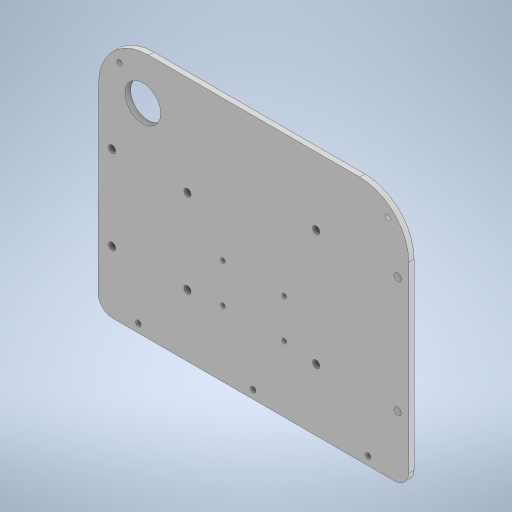
# Autodesk Inventor part: Final_Back_Cover_1
Saved by Autodesk Inventor 2023.5 (Build 275446020, 446B)
## iProperties
Created: 2025-04-13
Part Number: Final_Back_Cover_1
Material: Generic
Document SubType Name: Modeling
Designer: Lucky
Density: 1 g/cm^3
Appearance: Default
Author: Lucky
Autodesk Inventor part; units mm, degrees
ref_plane "YZ Plane" through (0, 0, 0) normal (1, 0, 0) x (0, 1, 0)
ref_plane "XZ Plane" through (0, 0, 0) normal (0, 1, 0) x (-1, 0, 0)
ref_plane "XY Plane" through (0, 0, 0) normal (0, 0, 1) x (1, 0, 0)
sketch "Sketch1" plane through (0, 0, 0) normal (0, 0, 1) x (1, 0, 0)
  arc A0 (-85.6258, 79.4796) -> (-116.0775, 49.6172) centre (-86.1702, 49.5773) ccw
  line L0 (-85.6258, 79.4796) -> (33.3305, 79.4959)
  arc A1 (63.2389, 49.5916) -> (33.3305, 79.4959) centre (33.3346, 49.5916) ccw
  line L1 (63.2389, -50.9075) -> (63.2389, 49.5916)
  line L2 (63.2389, 49.5916) -> (63.2389, -53.5021)
  line L3 (-116.0775, 49.6172) -> (-116.3855, -51.7391)
  line L4 (-116.0775, 49.6172) -> (-116.0775, -50.4074)
  arc A2 (-116.3855, -51.7391) -> (-106.0129, -63.5021) centre (-106.0129, -53.0473) ccw
  line L5 (-106.0129, -63.5021) -> (53.2389, -63.5021)
  arc A3 (53.2389, -63.5021) -> (63.2389, -53.5021) centre (53.2389, -53.5021) ccw
  arc A4 (-86.7039, 77.4795) -> (-114.0775, 49.6129) centre (-86.1702, 49.5773) ccw
  line L6 (-86.7039, 77.4795) -> (33.3308, 77.4959)
  arc A5 (61.2389, 49.5916) -> (33.3308, 77.4959) centre (33.3346, 49.5916) ccw
  line L7 (61.2389, 49.5916) -> (61.2389, -53.5021)
  arc A6 (53.2389, -61.5021) -> (61.2389, -53.5021) centre (53.2389, -53.5021) ccw
  line L8 (53.2389, -61.5021) -> (-106.0129, -61.5021)
  arc A7 (-114.3859, -51.8743) -> (-106.0129, -61.5021) centre (-106.0129, -53.0473) ccw
  line L9 (-114.3859, -51.8743) -> (-114.0775, 49.6129)
  line L10 (33.3308, 77.2959) -> (-85.6461, 77.2796)
  arc A8 (-85.6461, 77.2796) -> (-113.8775, 49.6124) centre (-86.1702, 49.5773) ccw
  line L11 (-113.8775, 49.6124) -> (-114.1859, -51.8886)
  arc A9 (-114.1859, -51.8886) -> (-106.0129, -61.3021) centre (-106.0129, -53.0473) ccw
  line L12 (-106.0129, -61.3021) -> (53.2389, -61.3021)
  arc A10 (53.2389, -61.3021) -> (61.0389, -53.5021) centre (53.2389, -53.5021) ccw
  line L13 (61.0389, -53.5021) -> (61.0389, 49.5916)
  arc A11 (61.0389, 49.5916) -> (33.3308, 77.2959) centre (33.3346, 49.5916) ccw
  circle A12 centre (-102.0292, 65.4774) radius 1.5
  circle A13 centre (49.2389, 65.498) radius 1.5
  circle A14 centre (-26.6496, -56.5021) radius 1.5
  circle A15 centre (-91.3999, -56.5021) radius 1.5
  circle A16 centre (38.2389, -56.5021) radius 1.5
  line L14 (-116.0775, -2.0021) -> (63.2389, -2.0021)
  line L15 (-43.7191, -2.0021) -> (-9.1191, -2.0021)
  line L16 (-9.1191, -2.0021) -> (-9.1191, -24.0021)
  line L17 (-9.1191, -24.0021) -> (-43.7191, -24.0021)
  line L18 (-43.7191, -24.0021) -> (-43.7191, -2.0021)
  circle A17 centre (-43.7191, -2.0021) radius 1.25
  circle A18 centre (-9.1191, -2.0021) radius 1.25
  circle A19 centre (-9.1191, -24.0021) radius 1.25
  circle A20 centre (-43.7191, -24.0021) radius 1.25
  line L19 (-63.7191, 9.7883) -> (-63.7191, -26.3021)
  circle A21 centre (-63.7191, 21.1979) radius 2
  circle A22 centre (-63.7191, -26.3021) radius 2
  line L20 (-63.7191, 21.1979) -> (-106.2191, 21.1979)
  line L21 (-63.7191, -26.3021) -> (-106.2191, -26.3021)
  line L22 (-106.2191, -26.3021) -> (-106.2191, 21.1979)
  circle A23 centre (-106.2191, 21.1979) radius 2
  circle A24 centre (-106.2191, -26.3021) radius 2
  line L23 (-63.7191, 9.7883) -> (-63.7191, 21.1979)
  line L24 (-109.1691, 24.1479) -> (-60.7691, 24.1479)
  line L25 (-60.7691, 24.1479) -> (-60.7691, 9.7883)
  line L26 (-60.7691, 9.7883) -> (-60.7691, -29.2521)
  line L27 (-60.7691, -29.2521) -> (-109.1691, -29.2521)
  line L28 (-109.1691, -29.2521) -> (-109.1691, 24.1479)
  line L29 (8.8809, 39.1979) -> (54.8809, 39.1979)
  line L30 (54.8809, 39.1979) -> (54.8809, -26.3021)
  line L31 (54.8809, -26.3021) -> (8.8809, -26.3021)
  line L32 (8.8809, -26.3021) -> (8.8809, 39.1979)
  circle A25 centre (8.8809, 39.1979) radius 2
  circle A26 centre (54.8809, 39.1979) radius 2
  circle A27 centre (8.8809, -26.3021) radius 2
  circle A28 centre (54.8809, -26.3021) radius 2
  circle A29 centre (-88.8693, 52.2792) radius 10
  point P0 (0, 0)
  point P1 (44.321, -53.9075)
  point P2 (51.321, -50.9075)
  point P3 (-9.1191, -13.0021)
  point P4 (-84.9691, -26.3021)
  dimension "d0" = 10
  dimension "d1" = 2
  dimension "d2" = 0.2
  dimension "d3" = 3
  dimension "d4" = 3
  dimension "d5" = 3
  dimension "d6" = 3
  dimension "d7" = 3
  dimension "d8" = 14
  dimension "d9" = 14
  dimension "d10" = 14
  dimension "d11" = 14
  dimension "d12" = 89.75
  dimension "d13" = 7
  dimension "d14" = 7
  dimension "d15" = 7
  dimension "d16" = 25
  dimension "d17" = 25
  dimension "d20" = 61.5
  dimension "d21" = 34.6
  dimension "d22" = 22
  dimension "d23" = 2.5
  dimension "d24" = 2.5
  dimension "d25" = 2.5
  dimension "d26" = 2.5
  dimension "d27" = 0
  dimension "d28" = 179.3164
  dimension "d29" = 72.358
  dimension "d32" = 20
  dimension "d33" = 47.5
  dimension "d34" = 4
  dimension "d35" = 4
  dimension "d36" = 42.5
  dimension "d37" = 4
  dimension "d38" = 4
  dimension "d39" = 48.4
  dimension "d51" = 46
  dimension "d52" = 65.5
  dimension "d53" = 18
  dimension "d54" = 35
  dimension "d55" = 35
  dimension "d56" = 4
  dimension "d57" = 4
  dimension "d58" = 4
  dimension "d59" = 4
  dimension "d62" = 20
  dimension "d63" = 25
  dimension "d64" = 25
  constraints: 66 end point, 29 centre point, 23 point on circle, 10 coincident, 6 horizontal, 5 perpendicular, 4 parallel, 4 point on line, 4 vertical, 2 midpoint, 2 tangent, 22 other
  measures "d0" radius of A3
  measures "d1" radial gap between concentric circles of A0 A4
  measures "d2" distance between parallel lines of L6 L10
  measures "d3" diameter of A12
  measures "d4" diameter of A13
  measures "d5" diameter of A14
  measures "d6" diameter of A15
  measures "d7" diameter of A16
  measures "d8" distance from line of A12.centre L0
  measures "d9" distance from line of L3 A12.centre
  measures "d10" distance from line of L0 A13.centre
  measures "d11" distance from line of L1 A13.centre
  measures "d12" distance from line of L3 A14.centre
  measures "d13" distance from line of L5 A14.centre
  measures "d14" distance from line of L5 A15.centre
  measures "d15" distance from line of L5 A16.centre
  measures "d16" distance from line of L3 A15.centre
  measures "d17" distance from line of L2 A16.centre
  measures "d20" distance between parallel lines of L5 L14
  measures "d21" distance of L16.end L17.end
  measures "d22" distance of L15.end L16.end
  measures "d23" diameter of A17
  measures "d24" diameter of A18
  measures "d25" diameter of A19
  measures "d26" diameter of A20
  measures "d27" distance between parallel lines of L15 L14
  measures "d28" distance between parallel lines of L1 L4
  measures "d29" distance between parallel lines of L1 L16
  measures "d32" distance between parallel lines of L18 L19
  measures "d33" distance of L19.end L20.start
  measures "d34" diameter of A21
  measures "d35" diameter of A22
  measures "d36" distance of L20.end L20.start
  measures "d37" diameter of A23
  measures "d38" diameter of A24
  measures "d39" distance between parallel lines of L28 L26
  measures "d51" distance of L30.end L31.end
  measures "d52" distance of L29.end L30.end
  measures "d53" distance from line of point (-9.119, -13.002) L32
  measures "d54" distance from line of L12 point (-84.969, -26.302)
  measures "d55" distance between parallel lines of L12 L31
  measures "d56" diameter of A25
  measures "d57" diameter of A26
  measures "d58" diameter of A27
  measures "d59" diameter of A28
  measures "d62" diameter of A29
  measures "d63" distance from line of L10 A29.centre
  measures "d64" distance from line of L11 A29.centre
extrude "Extrusion1" add sketch "Sketch1" along normal blind 3 contours L14 L28 L27 L26 A17 L18 A20 L17 A19 L16 A18 L32 A27 L31 A28 L30 L13 A10 L12 A9 L11 | L11 A8 L10 A11 L13 L14 L30 A26 L29 A25 L32 A18 A17 L26 L25 L24 L28 | L28 L24 L25 L26 L14 L19 L23 A21 L20 A23 L22 | L14 L22 A24 L21 A22 L19 L26 L27 L28 | L22 A23 L20 A21 L23 L19 L14 | L14 L19 A22 L21 A24 L22 | L30 A28 L31 A27 L32 L14 | L14 L32 A25 L29 A26 L30 | A24 L21 L22 | L22 L21 A24 | A23 L20 L22 | L22 L20 A23 | A26 L29 L30 | L30 L29 A26 | A28 L31 L30 | L30 L31 A28 | A22 L21 L19 | L19 L21 A22 | A18 L16 L14 | L14 A18 | A27 L31 L32 | L32 L31 A27 | A25 L29 L32 | L32 L29 A25 | A17 L14 | L14 L18 A17 | L23 L20 A21 | A21 L20 L23 | L16 A18 L14 | A18 L16 A19 L17 A20 L18 A17 L14 | L14 A17 L18 | A19 L17 L16 | L16 L17 A19 | A20 L17 L18 | L18 L17 A20 | A29
extrude "Extrusion2" cut sketch "Sketch1" along normal up to surface (3 mm away) contours A18 L16 L14 | L14 A18 | A17 L14 | L14 L18 A17 | L16 A18 L14 | L14 A17 L18 | A19 L17 L16 | L16 L17 A19 | A20 L17 L18 | L18 L17 A20
extrude "Extrusion3" cut sketch "Sketch1" along normal blind 3 contours A24 L21 L22 | L22 L21 A24 | A23 L20 L22 | L22 L20 A23 | A22 L21 L19 | L19 L21 A22 | L23 L20 A21 | A21 L20 L23
extrude "Extrusion5" cut sketch "Sketch1" along normal up to surface (3 mm away) contours A26 L29 L30 | L30 L29 A26 | A28 L31 L30 | L30 L31 A28 | A27 L31 L32 | L32 L31 A27 | A25 L29 L32 | L32 L29 A25
extrude "Extrusion6" cut sketch "Sketch1" along normal blind 3 contours A29
body "Solid1"
